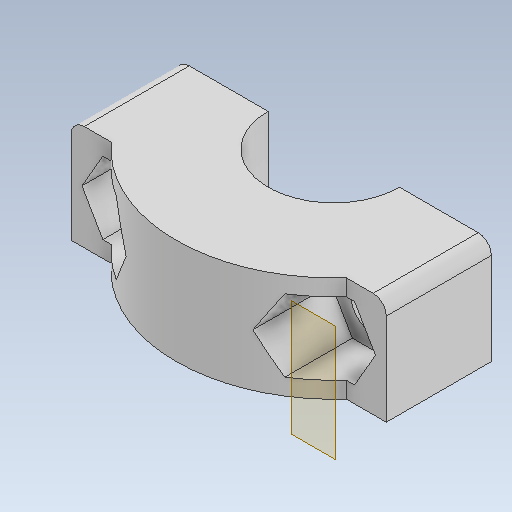
# Autodesk Inventor part: Bed Cable Harness Rod Clamp
Saved by Autodesk Inventor 2020 (Build 240168000, 168)
## iProperties
Created: 2019-12-21
Part Number: Bed Cable Harness Rod Clamp
Material: Generic
Document SubType Name: Modeling
Designer: pepd9
Density: 1 g/cm^3
Appearance: Default
Author: pepd9
Autodesk Inventor part; units mm, degrees
ref_plane "YZ Plane" through (0, 0, 0) normal (1, 0, 0) x (0, 1, 0)
ref_plane "XZ Plane" through (0, 0, 0) normal (0, 1, 0) x (-1, 0, 0)
ref_plane "XY Plane" through (0, 0, 0) normal (0, 0, 1) x (1, 0, 0)
sketch "Sketch1" plane through (0, 0, 0) normal (0, 1, 0) x (-1, 0, 0)
  circle A0 centre (5, -11.8206) radius 1.7 projected
  line L0 (9, -15) -> (9, -12) projected
  line L1 (1, -15) -> (3.5, -15) projected
  line L2 (1, -12) -> (1, -15) projected
  line L3 (1, -12) -> (-7, -12) projected
  line L4 (-7, -12) -> (-7, 0) projected
  line L5 (0, 0) -> (-7, 0) projected
  arc A1 (0, 0) -> (10, 0) centre (5, 0) ccw projected
  line L6 (17, 0) -> (10, 0) projected
  line L7 (17, 0) -> (17, -12) projected
  line L8 (17, -12) -> (9, -12) projected
  line L9 (-7, 12) -> (-7, 0)
  arc A2 (10, 0) -> (0, 0) centre (5, 0) ccw
  line L10 (17, 0) -> (17, 12)
  line L11 (-7, 12) -> (17, 12)
  line L12 (3.5, -14.5) -> (3.5, -15) projected
  line L13 (6.5, -15) -> (9, -15) projected
  line L14 (6.5, -15) -> (6.5, -14.5) projected
  line L15 (6.5, -14.5) -> (3.5, -14.5) projected
  constraints: 6 end point, 2 point on circle, 2 symmetric about line, 1 centre point, 1 perpendicular, 1 other
ref_plane "Work Plane1" through (-16, 8, -12) normal (0, 1, 0) x (0, 0, 1)
extrude "Extrusion1" add sketch "Sketch1" along normal up to surface (8 mm away) contours L6 A2 L5 L9 L11 L10
sketch "Sketch2" plane through (7, 0, 0) normal (0, 0, -1) x (-1, 0, 0)
  circle A0 centre (20, 4) radius 1.7 projected
  circle A1 centre (4, 4) radius 1.7 projected
  point P0 (7, 0)
sketch "Sketch3" plane through (-17, 8, 12) normal (0, 1, 0) x (1, 0, 0)
  line L0 (0, 0) -> (0, 12) projected
  line L1 (24, 0) -> (0, 0) projected
  line L2 (24, 12) -> (24, 0) projected
  line L3 (17, 12) -> (24, 12) projected
  arc A0 (7, 12) -> (17, 12) centre (12, 12) ccw projected
  line L4 (0, 12) -> (7, 12) projected
  line L5 (24, 12) -> (24, 0) projected
  circle A1 centre (12, 12) radius 12
  line L6 (0, 0) -> (0, 12) projected
  line L7 (24, 12) -> (0, 12)
  line L8 (0, 12) -> (0, 4)
  line L9 (0, 4) -> (24, 4)
  line L10 (24, 4) -> (24, 12)
  point P0 (24, 4)
  point P1 (20.9443, 4)
  point P2 (12, 0)
  point P3 (3.0557, 4)
  point P4 (0, 4)
  dimension "d2" = 8
  constraints: 8 end point, 2 parallel, 1 coincident, 1 horizontal, 1 perpendicular, 1 point on line, 3 other
  measures "d2" distance of L8.end L7.end
extrude "Extrusion2" cut sketch "Sketch3" against normal through all contours L0 L9 A1 L1 | A1 L9 L2 L1
hole "Hole1" at (3, 4, 0) at (-13, 4, 0) direction (0, 0, 1) diameter 3.4 end through all clearance for "Socket Head Cap Screw" size "M3" standard "Ansi Metric M Profile"
ref_plane "Work Plane2" through (3.9443, 8, 12) normal (0, 0, 1) x (1, 0, 0)
sketch "Sketch4" plane through (3.9443, 8, 12) normal (0, 0, 1) x (1, 0, 0)
  circle A0 centre (-16.9443, -4) radius 1.7 projected
  line L0 (-15.3566, -1.25) -> (-13.7688, -4)
  line L1 (-13.7688, -4) -> (-15.3566, -6.75)
  line L2 (-15.3566, -6.75) -> (-18.532, -6.75)
  line L3 (-18.532, -6.75) -> (-20.1197, -4)
  line L4 (-20.1197, -4) -> (-18.532, -1.25)
  line L5 (-18.532, -1.25) -> (-15.3566, -1.25)
  arc A1 (0, -5.4136) -> (0, -2.5864) centre (-0.9443, -4) ccw projected
  line L6 (0.6434, -1.25) -> (2.2312, -4)
  line L7 (2.2312, -4) -> (0.6434, -6.75)
  line L8 (0.6434, -6.75) -> (-2.532, -6.75)
  line L9 (-2.532, -6.75) -> (-4.1197, -4)
  line L10 (-4.1197, -4) -> (-2.532, -1.25)
  line L11 (-2.532, -1.25) -> (0.6434, -1.25)
  point P0 (-3.9443, -8)
  dimension "d13" = 5.5
  dimension "d14" = 5.5
  constraints: 24 end point, 2 coincident, 2 horizontal, 2 vertical alignment, 26 other
  measures "d13" distance between parallel lines of L2 L5
  measures "d14" distance between parallel lines of L8 L11
extrude "Extrusion3" cut sketch "Sketch4" against normal blind 7 contours A0 | L0 L1 L2 L3 L4 L5 | L6 L7 L8 L9 L10 L11
fillet "Fillet1" radius 1 2 edges at (-17, 8, 4) (7, 8, 4)
body "Solid1"
